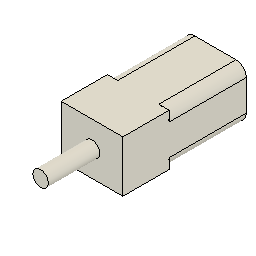
BuddyRover (Autodesk Fusion 360 archive; units mm, degrees)
design "n20"
Autodesk Fusion 360 part; units mm, degrees
sketch "草图1" plane through (0, 0, 0) normal (0, 0, 1) x (1, 0, 0)
  line L0 (6, -5) -> (-6, -5)
  line L1 (-6, -5) -> (-6, 5)
  line L2 (-6, 5) -> (6, 5)
  line L3 (6, 5) -> (6, -5)
  line L4 (6, -5) -> (-6, 5) construction
  line L5 (-6, -5) -> (6, 5) construction
  circle A0 centre (0, 0) radius 1.5
  dimension "d1" = 12
  dimension "d2" = 10
  dimension "d3" = 3
  constraint horizontal L0
  constraint perpendicular L0 L1
  constraint parallel L0 L2
  constraint parallel L1 L3
  constraint coincident L4 A0.centre
  constraint coincident L5 A0.centre
  constraint coincident A0.centre origin
  measures "d1" distance of L1.end L2.end
  measures "d2" distance of L0.end L1.end
  measures "d3" diameter of A0
extrude "拉伸1" add sketch "草图1" along normal blind 9 contours L0 L1 L2 L3 | A0 makes body 1
extrude "拉伸2" add sketch "草图1" against normal blind 15 separate body contours L0 L1 L2 L3 | A0 makes body 2
fillet "圆角1" radius 2 4 edges at (6, 5, -7.5) (-6, 5, -7.5) (6, -5, -7.5) (-6, -5, -7.5) on bodies 2
extrude "拉伸3" add sketch "草图1" along normal blind 19 contours A0 bodies 1 2
